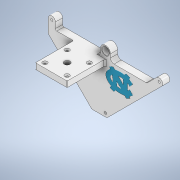
# Autodesk Inventor part: WinderBracket
Saved by Autodesk Inventor 2021 (Build 250183000, 183)
## iProperties
Created: 2020-03-15
Part Number: WinderBracket
Material: Generic
Document SubType Name: Modeling
Designer: elmar
Density: 1 g/cm^3
Appearance: Default
Author: elmar
Autodesk Inventor part; units mm, degrees
ref_plane "YZ Plane" through (0, 0, 0) normal (1, 0, 0) x (0, 1, 0)
ref_plane "XZ Plane" through (0, 0, 0) normal (0, 1, 0) x (-1, 0, 0)
ref_plane "XY Plane" through (0, 0, 0) normal (0, 0, 1) x (1, 0, 0)
sketch "Sketch1" plane through (0, 0, 0) normal (0, 0, 1) x (1, 0, 0)
  line L0 (-75, 0) -> (0, 75)
  line L1 (0, 75) -> (75, 0)
  line L2 (75, 0) -> (0, -75)
  line L3 (0, -75) -> (-75, 0)
  line L4 (-112, 0) -> (112, 0) projected
  line L5 (-80, 5) -> (80, 5)
  line L6 (80, 5) -> (80, -80)
  line L7 (80, -80) -> (-80, -80)
  line L8 (-80, -80) -> (-80, 5)
  line L9 (0, -111) -> (0, 106) projected
  line L10 (-70, 5) -> (70, 5)
  line L11 (70, 5) -> (70, -10)
  line L12 (70, -10) -> (-70, -10)
  line L13 (-70, -10) -> (-70, 5)
  circle A0 centre (75, 0) radius 5
  circle A1 centre (-75, 0) radius 5
  line L14 (-71.4645, 3.5355) -> (-57.9289, -10)
  line L15 (57.9289, -10) -> (71.4645, 3.5355)
  circle A2 centre (0, -75) radius 5
  line L16 (-78.5355, -3.5355) -> (-3.5355, -78.5355)
  line L17 (78.5355, -3.5355) -> (3.5355, -78.5355)
  line L18 (-80, -19.0878) -> (-19.0878, -80)
  point P0 (0, 0)
  point P1 (0, 0)
  point P2 (0, -80)
  point P3 (0, -10)
  point P4 (-70, 0)
  point P5 (-80, 0)
  point P6 (0, -80)
  dimension "d1" = 160
  dimension "d3" = 5
  dimension "d5" = 10
  dimension "d19" = 12.0326
  dimension "d64" = 106.066
  constraints: 34 end point, 10 tangent, 8 point on line, 6 parallel, 6 point on circle, 4 coincident, 4 perpendicular, 3 centre point, 2 horizontal, 2 midpoint, 1 equal radius, 9 other
  measures "d1" distance of L6.end L7.end
  measures "d3" distance from line of L7 L2.end
  measures "d5" distance between parallel lines of L12 L4
  measures "d19" distance between parallel lines of L18 L16
  measures "d64" distance of L2.end L0.start
extrude "Extrusion1" add sketch "Sketch1" along normal blind 10 contours L4 A1 L0 | L4 A1 L3 | L0 A1 L4 | L3 A1 L4 | A1 L13 L3 | L3 L13 L12 A2 L16 A1 | A1 L16 A2 L7 L18 L8 | L12 L9 A2 L3 | A2 L3 L9 | A2 L9 L3 | L9 L2 A2 | L15 L11 L4 | L4 L11 L2 L12 L15 | L12 L2 A2 L9 | A0 L4 L1 | L1 L4 A0 | A0 L11 L15 | L9 A2 L2 | A2 L2 L12 L11 A0 L17 | A0 L2 L11 | L4 L2 A0 | L4 A0 L2 | L11 L12 L2
hole "Hole1" at (-75, 0, 0) at (75, 0, 0) at (0, -75, 0) direction (0, 0, 1) diameter 3.2 end through all clearance for "Flat Head Machine Screw" size "M3" standard "Ansi Metric M Profile"
sketch "Sketch2" plane through (-57.0836, -10, 0) normal (0, 1, 0) x (1, 0, 0)
  circle A0 centre (34.5836, -41.15) radius 22.5
  line L0 (57.0836, 12.73) -> (57.0836, -76.38) projected
  line L1 (50.0836, -25.65) -> (50.0836, -56.65)
  line L2 (50.0836, -56.65) -> (19.0836, -56.65)
  line L3 (19.0836, -56.65) -> (19.0836, -25.65)
  line L4 (19.0836, -25.65) -> (50.0836, -25.65)
  line L5 (55.7336, -62.3) -> (13.4336, -62.3)
  line L6 (13.4336, -62.3) -> (13.4336, -20)
  line L7 (13.4336, -20) -> (55.7336, -20)
  line L8 (55.7336, -20) -> (55.7336, -62.3)
  line L9 (115.0126, -10) -> (-12.9164, -10) projected
  line L10 (12.4336, -63.3) -> (56.7336, -63.3)
  line L11 (56.7336, -63.3) -> (56.7336, -10)
  line L12 (56.7336, -10) -> (12.4336, -10)
  line L13 (12.4336, -10) -> (12.4336, -63.3)
  point P0 (57.0836, 0)
  point P1 (12.4336, -10)
  dimension "d15" = 45
  dimension "d16" = 31
  dimension "d17" = 42.3
  dimension "d18" = 10
  dimension "d21" = 1
  dimension "d22" = 1
  dimension "d23" = 1
  constraints: 24 end point, 2 coincident, 2 parallel, 2 vertical, 1 centre point, 1 horizontal, 1 perpendicular, 1 point on line, 1 tangent, 18 other
  measures "d15" diameter of A0
  measures "d16" distance of L1.end L2.end
  measures "d17" distance of L7.end L5.start
  measures "d18" distance between parallel lines of L9 L7
  measures "d21" distance between parallel lines of L8 L11
  measures "d22" distance between parallel lines of L5 L10
  measures "d23" distance between parallel lines of L6 L13
fillet "Fillet1" radius 2 4 edges at (-80, -19.0878, 5) (-19.0878, -80, 5) (57.9289, -10, 5) (-70, -10, 5)
extrude "Extrusion2" add sketch "Sketch2" against normal blind 8 contours L11 A0 L8 | A0 L8 L7 L6 L13 L9 L11 | L11 L10 A0 L5 L8 | L8 A0 L5 L6 L7 | A0 L7 L8 | L8 L5 A0 | L7 A0 | A0 L10 L5 | A0 L6 L7 | A0 L6 L13 | L5 L6 A0 | A0 L10 L13 L6 L5 | L1 L2 L3 L4
hole "Hole2" at (-7, -10, 25.65) at (-7, -10, 56.65) at (-38, -10, 56.65) at (-38, -10, 25.65) direction (0, -1, 0) diameter 3.2 end through all countersink diameter 6.3 countersink angle 90 clearance for "Flat Head Machine Screw" size "M3" standard "Ansi Metric M Profile"
sketch "Sketch3" plane through (-57.0836, -18, 0) normal (0, -1, 0) x (1, 0, 0)
  circle A0 centre (34.5836, 41.15) radius 11.5
  point P0 (57.0836, 0)
  dimension "d40" = 23
  constraints: 1 centre point, 1 coincident
  measures "d40" diameter of A0
hole "Hole3" at (-22.5, -10, 41.15) direction (0, -1, 0) diameter 8 end through all
extrude "Extrusion3" cut sketch "Sketch3" against normal blind 2.2
fillet "Fillet2" radius 1 2 edges at (-44.65, -14, 63.3) (-0.35, -14, 63.3)
fillet "Fillet3" radius 2 2 edges at (-44.65, -14, 10) (-0.35, -14, 10)
sketch "Sketch4" plane through (0, 0, 0) normal (0, 0, -1) x (-1, 0, 0)
  circle A0 centre (0, 0) radius 7
  line L0 (-7, 0) -> (-7, -10)
  line L1 (-57.1005, -10) -> (-1.65, -10) projected
  line L2 (7, 0) -> (7, -10)
  line L3 (43.65, -10) -> (1.35, -10) projected
  line L4 (-57.1005, -10) -> (68, -10) projected
  dimension "d45" = 14
  constraints: 4 end point, 2 point on circle, 2 point on line, 2 tangent, 1 centre point, 1 coincident, 1 parallel, 1 vertical
  measures "d45" diameter of A0
extrude "Extrusion4" add sketch "Sketch4" against normal up to surface (10 mm away)
hole "Hole4" at (0, 0, 0) direction (0, 0, 1) diameter 3 end through all countersink diameter 10 countersink angle 90
sketch "Sketch5" plane through (0, 0, 10) normal (0, 0, 1) x (1, 0, 0)
  point P0 (0, 0)
hole "Hole5" at (0, 0, 10) direction (0, 0, -1) diameter 3 end through all countersink diameter 10 countersink angle 90
fillet "Fillet4" radius 2 5 edges at (0, -1.5, 3.5) (-1.5, 0, 6.5) (1.5, 0, 6.5) (0, 5, 10) (0, -5, 0)
fillet "Fillet5" radius 5 2 edges at (7, -10, 5) (-7, -10, 5)
sketch "Sketch6" plane through (0, 0, 10) normal (0, 0, 1) x (1, 0, 0)
  spline S0 degree 3 poles (8.9522, -42.3911) (8.4412, -42.2534) (7.559, -42.0157) (6.8413, -41.5925) (5.9682, -41.5631) (6.1264, -41.2555) (6.3022, -41.0347) (6.6912, -40.5643) (7.2716, -39.8936) (7.6104, -39.2222) (8.2527, -38.6249) (7.8224, -38.3602) (7.4411, -38.0902) (5.9796, -37.2236) (3.8794, -35.6671) (1.6778, -32.9953) (0.712, -30.5704) (0.4161, -28.7909) (0.4165, -27.6211) (0.6983, -25.9119) (1.6018, -23.6351) (3.4938, -21.1515) (5.2051, -19.6858) (6.3449, -19.0002) (6.5458, -18.8399) (6.7932, -18.7422) (6.5551, -18.4149) (6.3819, -18.0088) (5.9935, -17.4008) (5.6331, -16.7925) (5.4152, -16.3702) (5.1914, -15.9278) (6.0292, -15.828) (6.7717, -15.3752) (7.6179, -15.0868) (8.107, -14.9202) knots 0 0 0 0 0.151269 0.26112 0.305797 0.318872 0.350882 0.395361 0.5004 0.605807 0.660491 0.682649 0.73638 0.810209 1.183666 1.521906 1.833015 1.953756 2.061528 2.182269 2.471804 2.785815 3.108418 3.147463 3.177276 3.191404 3.212778 3.267574 3.344153 3.421016 3.476597 3.499252 3.54442 3.653486 3.802871 3.802871 3.802871 3.802871
  line L0 (8.107, -14.9202) -> (10.8577, -13.8834)
  line L1 (10.8577, -13.8834) -> (11.9328, -15.0091)
  line L2 (11.9328, -15.0091) -> (13.0079, -16.1348)
  line L3 (13.0079, -16.1348) -> (13.8382, -15.9144)
  spline S1 degree 3 poles (13.8382, -15.9144) (14.9641, -15.7015) (17.4027, -15.2403) (21.1052, -15.1397) (23.9178, -15.2607) (25.606, -15.5652) (26.1763, -15.5967) (26.6098, -15.7363) (26.9059, -15.4091) (27.2663, -15.0044) (27.7622, -14.3264) (28.2149, -13.7461) (28.6118, -13.2042) (29.0778, -13.2483) (29.6414, -13.5318) (30.6048, -13.852) (31.7747, -14.3319) (32.9977, -14.7222) (33.7181, -15.1698) (34.3452, -15.2052) (34.3816, -15.4137) (34.3288, -15.5221) (34.1189, -15.8666) (33.6801, -16.4958) (33.4567, -17.1648) (32.88, -17.8165) (33.2819, -18.0001) (33.5957, -18.2145) (34.2995, -18.6074) (35.217, -19.184) (36.3072, -19.9702) (36.9752, -20.5525) (37.3094, -20.8438) knots 0 0 0 0 0.343332 0.743661 1.106598 1.189272 1.252956 1.283881 1.311918 1.372728 1.453762 1.557703 1.606182 1.63382 1.688377 1.796947 1.936026 2.071392 2.170234 2.211175 2.217893 2.230006 2.246003 2.340414 2.447103 2.499053 2.518346 2.561776 2.619952 2.756097 2.888977 3.02194 3.02194 3.02194 3.02194
  line L4 (37.3094, -20.8438) -> (38.062, -21.5264)
  line L5 (38.062, -21.5264) -> (36.9138, -22.7906)
  spline S2 degree 3 poles (36.9138, -22.7906) (36.6768, -23.0507) (36.1871, -23.5882) (35.4808, -24.358) (35.0102, -24.8665) (34.7946, -25.0995) knots 0 0 0 0 0.336837 0.696095 1 1 1 1
  line L6 (34.7946, -25.0995) -> (33.8236, -26.1442)
  line L7 (33.8236, -26.1442) -> (33.1505, -25.4711)
  spline S3 degree 3 poles (33.1505, -25.4711) (32.887, -25.2273) (32.3494, -24.7299) (31.7115, -24.3115) (30.886, -23.5895) (30.8582, -24.8962) (30.7272, -25.9663) (30.7065, -27.7684) (30.7809, -29.6967) (31.0576, -30.9253) (31.0657, -32.695) (32.0558, -31.8982) (32.7193, -31.3795) (33.3813, -30.7322) (33.7298, -30.3016) (33.8986, -30.1127) (34.5521, -29.8341) (35.4759, -31.9793) (36.5446, -32.9751) (38.5978, -34.5099) (37.1219, -35.7227) (35.9356, -36.7513) (34.7648, -37.4893) (34.174, -37.8618) knots 0 0 0 0 0.104297 0.212802 0.2714 0.334104 0.482887 0.665792 0.853074 1.038373 1.135241 1.197529 1.32276 1.428567 1.463858 1.490358 1.503312 1.669255 1.957254 2.117915 2.223455 2.425407 2.631136 2.631136 2.631136 2.631136
  line L8 (34.174, -37.8618) -> (33.3068, -38.3511)
  line L9 (33.3068, -38.3511) -> (33.8668, -39.3879)
  spline S4 degree 3 poles (33.8668, -39.3879) (33.9608, -39.5667) (34.1233, -39.8755) (34.2813, -40.2218) (34.4248, -40.599) (33.6625, -40.7324) (32.9697, -41.2439) (32.181, -41.587) (31.7251, -41.7854) knots 0 0 0 0 0.144061 0.248838 0.292599 0.397651 0.651775 1 1 1 1
  line L10 (31.7251, -41.7854) -> (29.16, -43.0096)
  line L11 (29.16, -43.0096) -> (28.016, -41.8153)
  line L12 (28.016, -41.8153) -> (26.8721, -40.6209)
  line L13 (26.8721, -40.6209) -> (25.7614, -40.8309)
  spline S5 degree 3 poles (25.7614, -40.8309) (24.6681, -40.9775) (22.361, -41.2868) (18.8621, -41.2344) (16.2734, -41.001) (14.727, -40.6919) (14.2618, -40.6555) (13.8873, -40.5298) (13.6291, -40.8798) (13.2823, -41.2986) (12.8532, -41.9351) (12.4351, -42.5719) (12.1104, -42.9839) (11.8476, -43.3973) (11.2064, -42.9853) (10.2806, -42.852) (9.4395, -42.5602) (8.9522, -42.3911) knots 0 0 0 0 0.330599 0.697654 1.045383 1.113109 1.165407 1.190974 1.218361 1.280057 1.363196 1.445638 1.505419 1.529749 1.574371 1.6842 1.835464 1.835464 1.835464 1.835464
  spline S6 degree 3 poles (21.6878, -35.2084) (21.5633, -35.0602) (21.1269, -34.5405) (20.199, -33.5591) (18.9285, -32.2192) (17.668, -30.8304) (16.5651, -29.8267) (16.1294, -29.1253) (15.5275, -28.8471) (15.815, -30.4736) (15.72, -31.2239) (15.6496, -31.7797) knots 0 0 0 0 0.058045 0.203562 0.405105 0.611302 0.769007 0.844077 0.864661 0.937712 1.146467 1.146467 1.146467 1.146467
  line L14 (15.6496, -31.7797) -> (15.6496, -34.8167)
  line L15 (15.6496, -34.8167) -> (16.895, -34.9821)
  spline S7 degree 3 poles (16.895, -34.9821) (17.637, -35.0588) (18.9798, -35.1976) (20.5891, -35.3703) (21.4385, -35.2451) (21.6878, -35.2084) knots 0 0 0 0 0.465962 0.84327 1 1 1 1
  spline S8 degree 3 poles (10.2148, -30.5835) (10.1987, -29.92) (10.1675, -28.6357) (9.9362, -26.7884) (9.6333, -25.6345) (9.4881, -25.0815) knots 0 0 0 0 0.199069 0.385331 0.556711 0.556711 0.556711 0.556711
  line L16 (9.4881, -25.0815) -> (9.2213, -24.2057)
  line L17 (9.2213, -24.2057) -> (8.3846, -24.9966)
  spline S9 degree 3 poles (8.3846, -24.9966) (7.808, -25.6074) (6.7646, -26.7127) (6.5618, -29.1454) (7.5947, -30.6695) (8.6815, -31.7297) (9.3147, -32.1218) (9.9703, -32.7515) (10.2218, -32.2515) (10.1785, -31.5909) (10.2005, -30.9813) (10.2148, -30.5835) knots 0 0 0 0 0.245949 0.445093 0.674299 0.78007 0.882469 0.942086 0.963499 1.026592 1.145168 1.145168 1.145168 1.145168
  spline S10 degree 3 poles (24.6522, -21.61) (24.3984, -21.5439) (23.6252, -21.3426) (22.1501, -21.3093) (20.9491, -21.3) (20.2829, -21.2949) knots 0 0 0 0 0.17869 0.544357 1 1 1 1
  line L18 (20.2829, -21.2949) -> (17.8968, -21.3376)
  line L19 (17.8968, -21.3376) -> (21.2641, -24.9208)
  line L20 (21.2641, -24.9208) -> (24.6314, -28.5041)
  line L21 (24.6314, -28.5041) -> (24.672, -25.0873)
  spline S11 degree 3 poles (24.672, -25.0873) (24.6755, -24.5109) (24.6816, -23.5182) (24.6943, -22.3582) (24.6616, -21.7762) (24.6522, -21.61) knots 0 0 0 0 0.497248 0.856442 1 1 1 1
  point P0 (7.5095, -41.9365)
  point P1 (6.4649, -41.5967)
  point P2 (6.0445, -41.4452)
  point P3 (6.0938, -41.3241)
  point P4 (6.2801, -41.0638)
  point P5 (6.5632, -40.7207)
  point P6 (7.2184, -39.8997)
  point P7 (7.8311, -39.042)
  point P8 (8.102, -38.567)
  point P9 (7.9313, -38.4257)
  point P10 (7.4839, -38.1281)
  point P11 (6.8566, -37.7388)
  point P12 (3.8874, -35.4737)
  point P13 (1.7777, -32.8299)
  point P14 (0.6315, -29.9376)
  point P15 (0.4441, -28.7448)
  point P16 (0.4441, -27.6671)
  point P17 (0.6315, -26.4743)
  point P18 (1.6818, -23.7762)
  point P19 (3.5521, -21.2539)
  point P20 (6.0323, -19.1909)
  point P21 (6.3609, -18.9801)
  point P22 (6.6115, -18.8184)
  point P23 (6.7297, -18.741)
  point P24 (6.6522, -18.5418)
  point P25 (6.3899, -18.0608)
  point P26 (5.9994, -17.402)
  point P27 (5.6106, -16.7389)
  point P28 (5.3528, -16.2465)
  point P29 (5.2818, -16.0314)
  point P30 (5.6962, -15.8518)
  point P31 (6.7112, -15.4526)
  point P32 (17.2264, -15.3595)
  point P33 (21.2259, -15.1855)
  point P34 (24.8467, -15.4352)
  point P35 (25.6644, -15.5569)
  point P36 (26.2953, -15.6437)
  point P37 (26.6028, -15.6768)
  point P38 (26.8217, -15.5018)
  point P39 (27.2207, -15.0428)
  point P40 (27.7132, -14.3993)
  point P41 (28.3413, -13.5711)
  point P42 (28.6998, -13.2448)
  point P43 (28.9761, -13.2499)
  point P44 (29.4861, -13.4438)
  point P45 (30.5012, -13.8289)
  point P46 (31.8017, -14.3219)
  point P47 (33.0659, -14.8058)
  point P48 (33.9859, -15.1671)
  point P49 (34.3625, -15.3276)
  point P50 (34.3732, -15.3939)
  point P51 (34.3337, -15.5084)
  point P52 (34.2526, -15.6463)
  point P53 (33.7554, -16.4489)
  point P54 (33.2392, -17.3826)
  point P55 (33.0297, -17.858)
  point P56 (33.1919, -17.9625)
  point P57 (33.5642, -18.1861)
  point P58 (34.066, -18.4805)
  point P59 (35.2198, -19.2031)
  point P60 (36.2937, -19.9857)
  point P61 (36.2024, -23.5705)
  point P62 (35.4411, -24.4)
  point P63 (32.369, -24.7804)
  point P64 (31.5067, -24.1218)
  point P65 (30.9996, -23.8283)
  point P66 (30.8628, -24.4403)
  point P67 (30.758, -25.9244)
  point P68 (30.7224, -27.7531)
  point P69 (30.8241, -29.6232)
  point P70 (31.0408, -31.4634)
  point P71 (31.2703, -32.4045)
  point P72 (31.8114, -32.0959)
  point P73 (32.7784, -31.3002)
  point P74 (33.5243, -30.5498)
  point P75 (33.7517, -30.2798)
  point P76 (33.9456, -30.0993)
  point P77 (34.0642, -30.0472)
  point P78 (35.2199, -31.238)
  point P79 (37.1295, -33.3939)
  point P80 (38.1371, -34.6452)
  point P81 (37.4563, -35.4517)
  point P82 (35.8882, -36.7243)
  point P83 (34.1395, -39.9195)
  point P84 (34.3161, -40.3165)
  point P85 (34.3585, -40.4929)
  point P86 (33.9726, -40.6951)
  point P87 (33.0265, -41.1594)
  point P88 (22.4753, -41.1933)
  point P89 (18.8048, -41.1866)
  point P90 (15.3477, -40.8119)
  point P91 (14.6802, -40.6974)
  point P92 (14.1637, -40.6156)
  point P93 (13.9099, -40.5844)
  point P94 (13.7084, -40.7698)
  point P95 (13.3288, -41.2562)
  point P96 (12.8532, -41.9381)
  point P97 (12.3886, -42.6191)
  point P98 (12.0374, -43.1029)
  point P99 (11.8758, -43.2848)
  point P100 (11.4475, -43.1596)
  point P101 (10.3972, -42.8386)
  point P102 (21.312, -34.766)
  point P103 (20.327, -33.6949)
  point P104 (18.9459, -32.2271)
  point P105 (17.5268, -30.7311)
  point P106 (16.4422, -29.5863)
  point P107 (15.9268, -29.0404)
  point P108 (15.7351, -28.9654)
  point P109 (15.6616, -29.6922)
  point P110 (19.1254, -35.2143)
  point P111 (20.9391, -35.2999)
  point P112 (10.1321, -28.5945)
  point P113 (9.8882, -26.7479)
  point P114 (6.9326, -26.9817)
  point P115 (6.7777, -28.9671)
  point P116 (7.9198, -30.9544)
  point P117 (8.6834, -31.6863)
  point P118 (9.4941, -32.3118)
  point P119 (10.0266, -32.5799)
  point P120 (10.1385, -32.3973)
  point P121 (10.1977, -31.7691)
  point P122 (23.8876, -21.4315)
  point P123 (22.2849, -21.3159)
  point P124 (24.6842, -23.3579)
  point P125 (24.6771, -22.1087)
  point P126 (21.6878, -35.2084)
  point P127 (25.755, -40.8318)
  point P128 (31.7251, -41.7854)
  point P129 (34.174, -37.8618)
  point P130 (33.1505, -25.4711)
  point P131 (36.9124, -22.7921)
  point P132 (13.8383, -15.9143)
  point P133 (8.107, -14.9202)
  point P134 (8.3824, -24.9989)
  constraints: 44 end point, 150 other
extrude "Extrusion5" cut sketch "Sketch6" against normal blind 0.4
extrude "Extrusion6" add sketch "Sketch6" against normal blind 0.4 separate body
sketch "Sketch7" plane through (0, 0, 0) normal (0, 0, -1) x (-1, 0, 0)
  circle A0 centre (-75, 0) radius 1.6 projected
  line L0 (-76.6166, 2.8) -> (-73.3834, 2.8)
  line L1 (-73.3834, 2.8) -> (-71.7668, 0)
  line L2 (-71.7668, 0) -> (-73.3834, -2.8)
  line L3 (-73.3834, -2.8) -> (-76.6166, -2.8)
  line L4 (-76.6166, -2.8) -> (-78.2332, 0)
  line L5 (-78.2332, 0) -> (-76.6166, 2.8)
  circle A1 centre (75, 0) radius 1.6 projected
  line L6 (73.3834, 2.8) -> (76.6166, 2.8)
  line L7 (76.6166, 2.8) -> (78.2332, 0)
  line L8 (78.2332, 0) -> (76.6166, -2.8)
  line L9 (76.6166, -2.8) -> (73.3834, -2.8)
  line L10 (73.3834, -2.8) -> (71.7668, 0)
  line L11 (71.7668, 0) -> (73.3834, 2.8)
  circle A2 centre (0, -75) radius 1.6 projected
  line L12 (-1.6166, -72.2) -> (1.6166, -72.2)
  line L13 (1.6166, -72.2) -> (3.2332, -75)
  line L14 (3.2332, -75) -> (1.6166, -77.8)
  line L15 (1.6166, -77.8) -> (-1.6166, -77.8)
  line L16 (-1.6166, -77.8) -> (-3.2332, -75)
  line L17 (-3.2332, -75) -> (-1.6166, -72.2)
  point P0 (0, 0)
  dimension "d69" = 5.6
  constraints: 36 end point, 3 coincident, 3 horizontal, 2 parallel, 39 other
  measures "d69" distance between parallel lines of L12 L15
extrude "Extrusion7" cut sketch "Sketch7" against normal blind 2.6 contours A0 | L0 L1 L2 L3 L4 L5 | A1 | L6 L7 L8 L9 L10 L11 | A2 | L12 L13 L14 L15 L16 L17 bodies 1
sketch "Sketch8" plane through (0, 0, 0) normal (0, 0, -1) x (-1, 0, 0)
  circle A0 centre (0, 0) radius 1.5 projected
  circle A1 centre (0, 0) radius 5
  dimension "d80" = 10
  constraints: 1 centre point, 1 coincident
  measures "d80" diameter of A1
extrude "Extrusion8" cut sketch "Sketch8" against normal through all contours A0 | A1 bodies 1
equation "\"d1\" = BasePlateWidth"
equation "\"d3\" = MountHoleToSideDistance"
equation "\"d19\" = d2"
equation "\"d6\" = d5"
equation "\"d8\" = M3HoleDiameter"
equation "\"d26\" = M3HoleDiameter"
equation "\"d28\" = M3CounterSinkDiameter"
equation "\"d67\" = d65"
equation "\"SupportHoleDistance\" = 67.96736"
equation "\"BasePlateWidth\" = 160"
equation "\"MountHoleToSideDistance\" = 5"
equation "\"d2\" = 12.032642"
equation "\"M3HoleDiameter\" = 3.2"
equation "\"M3CounterSinkDiameter\" = 6.3"
equation "\"d65\" = 0.4"
